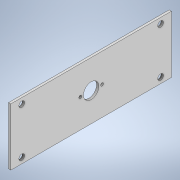
# Autodesk Inventor part: Motorhalterplatte
Saved by Autodesk Inventor 2022 (Build 260153000, 153)
## iProperties
Created: 2022-03-17
Part Number: Motorhalterplatte
Material: Generisch
Document SubType Name: Modeling
Designer: 123St
Density: 1 g/cm^3
Appearance: Vorgabe
Author: 123St
Autodesk Inventor part; units mm, degrees
ref_plane "YZ Plane" through (0, 0, 0) normal (1, 0, 0) x (0, 1, 0)
ref_plane "XZ Plane" through (0, 0, 0) normal (0, 1, 0) x (-1, 0, 0)
ref_plane "XY Plane" through (0, 0, 0) normal (0, 0, 1) x (1, 0, 0)
sketch "Skizze1" plane through (0, 0, 0) normal (1, 0, 0) x (0, 1, 0)
  line L0 (25, 70) -> (-25, 70)
  line L1 (-25, 70) -> (-25, -70)
  line L2 (-25, -70) -> (25, -70)
  line L3 (25, -70) -> (25, 70)
  line L4 (25, 70) -> (-25, -70) construction
  line L5 (-25, 70) -> (25, -70) construction
  point P0 (0, 0)
  dimension "d0" = 140
  dimension "d1" = 50
  constraints: 12 end point, 2 midpoint, 2 parallel, 1 horizontal, 1 perpendicular
  measures "d0" distance of L2.end L0.start
  measures "d1" distance of L1.end L2.end
extrude "Extrusion1" add sketch "Skizze1" along normal blind 2
sketch "Skizze2" plane through (2, 0, 0) normal (1, 0, 0) x (0, 0, -1)
  circle A0 centre (-60.5, 20) radius 2.5
  circle A1 centre (-60.5, -20) radius 2.5
  circle A2 centre (60.5, 20) radius 2.5
  circle A3 centre (60.5, -20) radius 2.5
  point P0 (0, 0)
  dimension "d4" = 5
  dimension "d5" = 5
  dimension "d6" = 5
  dimension "d7" = 5
  dimension "d8" = 121
  dimension "d9" = 60.5
  dimension "d10" = 121
  dimension "d11" = 60.5
  dimension "d12" = 40
  dimension "d13" = 20
  constraints: 4 centre point
  measures "d4" diameter of A0
  measures "d5" diameter of A1
  measures "d6" diameter of A2
  measures "d7" diameter of A3
  measures "d8" distance of A0.centre A2.centre
  measures "d9" horizontal distance of point (0, 0) A0.centre
  measures "d10" distance of A3.centre A1.centre
  measures "d11" horizontal distance of point (0, 0) A1.centre
  measures "d12" distance of A1.centre A0.centre
  measures "d13" vertical distance of point (0, 0) A1.centre
extrude "Extrusion2" cut sketch "Skizze2" against normal blind 2
sketch "Skizze3" plane through (2, 0, 0) normal (1, 0, 0) x (0, 0, -1)
  circle A0 centre (0, 0) radius 6.75
  circle A1 centre (9.5, 0) radius 1.25
  circle A2 centre (-9.5, 0) radius 1.25
  dimension "d16" = 2.5
  dimension "d17" = 2.5
  dimension "d18" = 13.5
  dimension "d19" = 19
  dimension "d20" = 9.5
  constraints: 3 centre point, 1 coincident
  measures "d16" diameter of A1
  measures "d17" diameter of A2
  measures "d18" diameter of A0
  measures "d19" distance of A2.centre A1.centre
  measures "d20" distance of point (0, 0) A1.centre
extrude "Extrusion3" cut sketch "Skizze3" against normal blind 2
equation "\"d9\" = 0.5 * d8"
equation "\"d10\" = d8"
equation "\"d11\" = 0.5 * d10"
equation "\"d20\" = 0.5 * d19"
